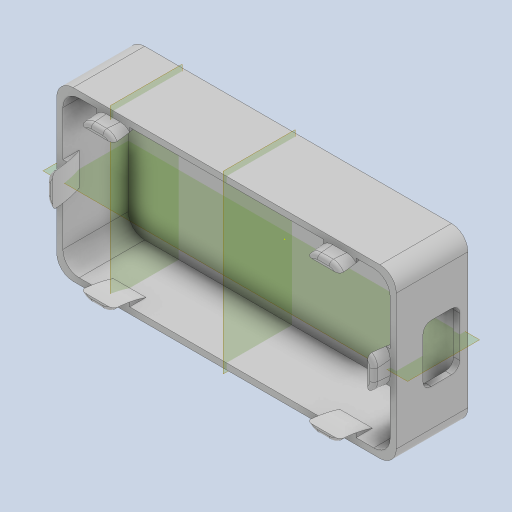
# Autodesk Inventor part: caja_superior
Saved by Autodesk Inventor 2024 (Build 280153000, 153)
## iProperties
Created: 2025-12-14
Part Number: caja_superior
Material: Genérico
Document SubType Name: Modeling
Designer: ANDRES
Density: 1 g/cm^3
Appearance: Valor por defecto
Author: ANDRES
Autodesk Inventor part; units mm, degrees
ref_plane "YZ Plane" through (0, 0, 0) normal (1, 0, 0) x (0, 1, 0)
ref_plane "XZ Plane" through (0, 0, 0) normal (0, 1, 0) x (-1, 0, 0)
ref_plane "XY Plane" through (0, 0, 0) normal (0, 0, 1) x (1, 0, 0)
sketch "Boceto1" plane through (0, 0, 0) normal (0, 0, 1) x (1, 0, 0)
  line L0 (-39.75, 22.25) -> (43.25, 22.25)
  line L1 (43.25, 22.25) -> (43.25, -18.75)
  line L2 (43.25, -18.75) -> (-39.75, -18.75)
  line L3 (-39.75, -18.75) -> (-39.75, 22.25)
  dimension "ancho" = 41
  dimension "largo" = 83
  constraints: 8 end point, 2 parallel, 1 horizontal, 1 perpendicular
  measures "ancho" distance of L0.end L1.end
  measures "largo" distance between parallel lines of L3 L1
extrude "Extrusión1" add sketch "Boceto1" along normal blind 1.5
sketch "Boceto2" plane through (0, 0, 1.5) normal (0, 0, 1) x (1, 0, 0)
  line L0 (-39.75, -18.75) -> (-39.75, 22.25) projected
  line L1 (-39.75, 22.25) -> (43.25, 22.25) projected
  line L2 (43.25, 22.25) -> (43.25, -18.75) projected
  line L3 (43.25, -18.75) -> (-39.75, -18.75) projected
  line L4 (41.75, 20.75) -> (-38.25, 20.75)
  line L5 (-38.25, 20.75) -> (-38.25, -17.25)
  line L6 (-38.25, -17.25) -> (41.75, -17.25)
  line L7 (41.75, -17.25) -> (41.75, 20.75)
  point P0 (0, 0)
  dimension "d5" = 1.5
  constraints: 8 end point, 3 other
  measures "d5" distance between parallel lines of L1 L4
extrude "Extrusión2" add sketch "Boceto2" along normal blind 16
sketch "Boceto3" plane through (43.25, -18.75, 0) normal (1, 0, 0) x (0, 0, -1)
  line L0 (-11, 27) -> (-2, 27)
  line L1 (-2, 27) -> (-2, 13)
  line L2 (-2, 13) -> (-11, 13)
  line L3 (-11, 13) -> (-11, 27)
  line L4 (-11, 27) -> (-2, 13) construction
  line L5 (-2, 27) -> (-11, 13) construction
  line L6 (0, 41) -> (-17.5, 41) projected
  line L7 (0, 0) -> (-17.5, 0) projected
  point P0 (0, 18.75)
  point P1 (-6.5, 20)
  point P2 (-6.5, 13)
  dimension "d8" = 14
  dimension "d9" = 9
  dimension "d10" = 21
  dimension "d11" = 14
  dimension "d12" = 13
  dimension "d13" = 2
  constraints: 12 end point, 3 midpoint, 2 parallel, 1 horizontal, 1 perpendicular
  measures "d8" distance between parallel lines of L2 L0
  measures "d9" distance between parallel lines of L1 L3
  measures "d10" distance from line of L6 point (-6.5, 20)
  measures "d11" distance between parallel lines of L6 L0
  measures "d12" distance from line of L7 point (-6.5, 13)
  measures "d13" distance from line of point (0, 18.75) L1
extrude "Extrusión3" cut sketch "Boceto3" against normal blind 16
fillet "Empalme1" radius 2 4 edges at (42.5, -5.75, 2) (42.5, 8.25, 2) (42.5, 8.25, 11) (42.5, -5.75, 11)
ref_plane "Plano de trabajo1" through (1.75, -17.25, 1.5) normal (-1, 0, 0) x (0, 0, 1)
ref_plane "Plano de trabajo2" through (-38.25, 1.75, 1.5) normal (0, -1, 0) x (1, 0, 0)
sketch "Boceto4" plane through (41.75, -17.25, 1.5) normal (-1, 0, 0) x (0, 0, 1)
  arc A0 (2.5, 25.5) -> (0.5, 23.5) centre (2.5, 23.5) ccw projected
  line L0 (0.5, 23.5) -> (0.5, 13.5) projected
  arc A1 (0.5, 13.5) -> (2.5, 11.5) centre (2.5, 13.5) ccw projected
  line L1 (2.5, 11.5) -> (7.5, 11.5) projected
  arc A2 (7.5, 11.5) -> (9.5, 13.5) centre (7.5, 13.5) ccw projected
  line L2 (9.5, 13.5) -> (9.5, 23.5) projected
  arc A3 (9.5, 23.5) -> (7.5, 25.5) centre (7.5, 23.5) ccw projected
  line L3 (7.5, 25.5) -> (2.5, 25.5) projected
  line L4 (0, 0) -> (16, 0) projected
  line L5 (16, 38) -> (16, 0) projected
  line L6 (16, 38) -> (0, 38) projected
  line L7 (0, 0) -> (0, 38) projected
  line L8 (16, 0) -> (16, -1.5) projected
  line L9 (16, -1.5) -> (-1.5, -1.5) projected
  line L10 (-1.5, -1.5) -> (-1.5, 39.5) projected
  line L11 (-1.5, 39.5) -> (16, 39.5) projected
  line L12 (16, 39.5) -> (16, 38) projected
  line L13 (20, 38) -> (12, 38)
  arc A4 (12, 38) -> (20, 36.5) centre (21.4775, 66.4636) ccw
  line L14 (20, 38) -> (20, 36.5)
  point P0 (-1.5, 17.25)
  point P1 (11.479, 40.458)
  point P2 (12, 38)
  dimension "d24" = 8
  dimension "d25" = 30
  dimension "d26" = 1.5
  constraints: 4 end point, 2 point on circle, 1 centre point, 1 coincident, 1 horizontal, 1 horizontal alignment, 1 midpoint, 1 vertical
  measures "d24" distance of L13.start L13.end
  measures "d25" radius of A4
  measures "d26" distance of L13.start L14.end
extrude "Extrusión4" [suppressed]
fillet "Empalme2" [suppressed]
mirror "Simetría1" [suppressed]
mirror "Simetría2" [suppressed]
fillet "Empalme3" radius 4 8 edges at (41.75, -17.25, 9.5) (41.75, 20.75, 9.5) (-38.25, 20.75, 9.5) (-38.25, -17.25, 9.5) (-39.75, -18.75, 8.75) (43.25, -18.75, 8.75) (43.25, 22.25, 8.75) (-39.75, 22.25, 8.75)
sketch "Boceto5" plane through (0, 0, 1.5) normal (0, 0, 1) x (1, 0, 0)
  point P0 (0, 0)
sketch "Boceto6" plane through (1.75, -17.25, 1.5) normal (-1, 0, 0) x (0, 0, 1)
  line L0 (16, 0) -> (16, -1.5) projected
  line L1 (16, -1.5) -> (-1.5, -1.5) projected
  line L2 (-1.5, -1.5) -> (-1.5, 39.5) projected
  line L3 (-1.5, 39.5) -> (16, 39.5) projected
  line L4 (16, 39.5) -> (16, 38) projected
  line L5 (16, 38) -> (0, 38) projected
  line L6 (0, 38) -> (0, 0) projected
  line L7 (0, 0) -> (16, 0) projected
  line L8 (12, 38) -> (20, 38)
  line L9 (20, 38) -> (20, 36.5)
  arc A0 (12, 38) -> (20, 36.5) centre (21.4775, 66.4636) ccw
  point P0 (-1.5, 17.25)
  point P1 (16, 38)
  point P2 (16, 38)
  point P3 (12, 38)
  dimension "d31" = 1.5
  dimension "d32" = 8
  dimension "d33" = 30
  constraints: 4 end point, 2 coincident, 2 point on circle, 1 centre point, 1 horizontal, 1 midpoint, 1 vertical
  measures "d31" distance of L8.end L9.end
  measures "d32" distance of L8.start L8.end
  measures "d33" radius of A0
extrude "Extrusión5" [suppressed]
fillet "Empalme4" [suppressed]
fillet "Empalme5" [suppressed]
mirror "Simetría3" [suppressed]
sketch "Boceto7" plane through (-38.25, 1.75, 1.5) normal (0, -1, 0) x (1, 0, 0)
  line L0 (80, 16) -> (81.5, 16) projected
  line L1 (81.5, 16) -> (81.5, 9.5) projected
  line L2 (81.5, 9.5) -> (80, 9.5) projected
  line L3 (80, 9.5) -> (80, 16) projected
  line L4 (80, 0) -> (80, 0.5) projected
  line L5 (80, 0.5) -> (81.5, 0.5) projected
  line L6 (81.5, 0.5) -> (81.5, -1.5) projected
  line L7 (81.5, -1.5) -> (-1.5, -1.5) projected
  line L8 (-1.5, -1.5) -> (-1.5, 16) projected
  line L9 (-1.5, 16) -> (0, 16) projected
  line L10 (0, 16) -> (0, 0) projected
  line L11 (0, 0) -> (80, 0) projected
  line L12 (80, 12) -> (80, 20)
  line L13 (80, 20) -> (78.5, 20)
  arc A0 (78.5, 20) -> (80, 12) centre (108.4636, 21.4775) ccw
  point P0 (38.25, -1.5)
  point P1 (80, 12)
  dimension "d38" = 1.5
  dimension "d39" = 8
  dimension "d40" = 30
  constraints: 4 end point, 2 coincident, 2 point on circle, 1 centre point, 1 midpoint, 1 perpendicular, 1 vertical
  measures "d38" distance of L12.end L13.end
  measures "d39" distance of L12.start L12.end
  measures "d40" radius of A0
extrude "Extrusión6" add sketch "Boceto7" along normal mid plane 8 contours L3 A0 L13 L12
fillet "Empalme6" radius 3 2 edges at (41.75, -2.25, 19.5) (41.75, 5.75, 19.5)
fillet "Empalme7" radius 1 3 edges at (41.3482, -1.1513, 21.5) (41.3482, 4.6513, 21.5) (41.75, 1.75, 21.5)
mirror "Simetría4" about plane through (1.75, -17.25, 1.5) normal (-1, 0, 0) of "Extrusión6", "Empalme7", "Empalme6"
ref_plane "Plano de trabajo3" through (-25.9167, -17.25, 1.5) normal (-1, 0, 0) x (0, 0, 1)
sketch "Boceto8" plane through (-25.9167, -17.25, 1.5) normal (-1, 0, 0) x (0, 0, 1)
  line L0 (16, -13.8135) -> (16, -15.3135)
  line L1 (16, -15.3135) -> (-1.5, -15.3135)
  line L2 (-1.5, -15.3135) -> (-1.5, 39.5)
  line L3 (-1.5, 39.5) -> (16, 39.5)
  line L4 (16, 39.5) -> (16, 38)
  line L5 (16, 38) -> (0, 38)
  line L6 (0, 38) -> (0, -13.8135)
  line L7 (0, -13.8135) -> (16, -13.8135)
  line L8 (12, 38) -> (20, 38)
  line L9 (20, 38) -> (20, 36.5)
  arc A0 (12, 38) -> (20, 36.5) centre (21.4775, 66.4636) ccw
  line L10 (-1.5, 39.5) -> (16, 39.5) projected
  line L11 (16, 39.5) -> (16, 38) projected
  line L12 (16, 38) -> (0, 38) projected
  line L13 (0, 38) -> (0, 0) projected
  line L14 (0, 0) -> (16, 0) projected
  line L15 (16, 0) -> (16, -1.5) projected
  line L16 (16, -1.5) -> (-1.5, -1.5) projected
  line L17 (-1.5, -1.5) -> (-1.5, 39.5) projected
  point P0 (-1.5, 17.25)
  point P1 (25.1174, 2.4365)
  point P2 (16, 38)
  point P3 (42.6174, 22.1865)
  point P4 (38.6174, 22.1865)
  point P5 (16, 38)
  point P6 (12, 38)
  dimension "d46" = 1.5
  dimension "d47" = 8
  dimension "d48" = 30
  constraints: 18 end point, 2 coincident, 2 point on circle, 1 centre point, 1 horizontal, 1 midpoint, 1 vertical, 3 other
  measures "d46" distance of L8.end L9.end
  measures "d47" distance of L8.start L8.end
  measures "d48" radius of A0
extrude "Extrusión7" add sketch "Boceto8" along normal mid plane 8 contours L5 L8 L9 A0
fillet "Empalme8" radius 3 2 edges at (-21.9167, 20.75, 19.5) (-29.9167, 20.75, 19.5)
fillet "Empalme9" radius 1 3 edges at (-23.0154, 20.3482, 21.5) (-28.818, 20.3482, 21.5) (-25.9167, 20.75, 21.5)
mirror "Simetría5" about plane through (-38.25, 1.75, 1.5) normal (0, -1, 0) of "Extrusión7", "Empalme9", "Empalme8"
mirror "Simetría6" about plane through (1.75, -17.25, 1.5) normal (-1, 0, 0) of "Extrusión7", "Empalme9", "Empalme8", "Simetría5"
equation "\"d5\" = espesor"
equation "\"d26\" = espesor"
equation "\"d31\" = espesor"
equation "\"d38\" = espesor"
equation "\"d46\" = d49"
equation "\"d18\" = 0.5 * ancho - espesor"
equation "\"d45\" = 0.333333 * largo"
equation "\"espesor\" = 1.5"
equation "\"d49\" = 1.5"
